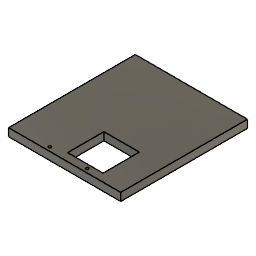
Full (Autodesk Fusion 360 archive; units mm, degrees)
design "rightside"
Autodesk Fusion 360 part; units mm, degrees
sketch "Skizze1" plane through (0, 0, 0) normal (0, 0, 1) x (1, 0, 0)
  line L0 (0, 0) -> (127, 0)
  line L1 (127, 0) -> (127, 143.5)
  line L2 (127, 143.5) -> (0, 143.5)
  line L3 (0, 143.5) -> (0, 0)
  line L4 (98, 50) -> (58, 50)
  line L5 (58, 50) -> (58, 9)
  line L6 (58, 9) -> (98, 9)
  line L7 (98, 9) -> (98, 50)
  circle A0 centre (84.6667, 4.5) radius 1.5
  circle A1 centre (42.3337, 4.5) radius 1.5
  dimension "d1" = 127
  dimension "d2" = 143.5
  dimension "d3" = 40
  dimension "d4" = 29
  dimension "d5" = 50
  dimension "d6" = 41
  dimension "d7" = 3
  dimension "d8" = 4.5
  dimension "d9" = 42.3333
  dimension "d10" = 3
  constraint horizontal L0
  constraint vertical L1
  constraint horizontal L2
  constraint vertical L3
  constraint coincident L0.start L3.end
  constraint perpendicular L3 L4
  constraint perpendicular L4 L5
  constraint perpendicular L5 L6
  constraint perpendicular L4 L7
  measures "d1" distance of L0.start L0.end
  measures "d2" distance of L0.start L2.end
  measures "d3" distance of L4.start L4.end
  measures "d4" distance of L1 L4.start
  measures "d5" distance of L0 L4
  measures "d6" distance of L4.end L5.end
  measures "d7" diameter of A0
  measures "d8" distance of L0 A0.centre
  measures "d9" distance of L1 A0.centre
  measures "d10" diameter of A1
extrude "Extrusion1" add sketch "Skizze1" along normal blind 9
equation "d5 = 41 mm + 9 mm"
equation "d8 = ( 9 / 2 ) * 1 mm"
equation "d9 = ( 127 / 3 ) * 1 mm"

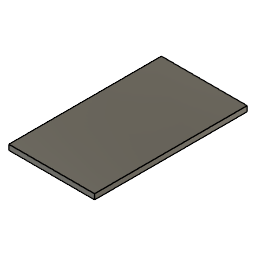
design "Top"
Autodesk Fusion 360 part; units mm, degrees
sketch "Skizze1" plane through (0, 0, 0) normal (0, 0, 1) x (1, 0, 0)
  line L0 (0, 0) -> (145, 0)
  line L1 (145, 0) -> (145, 258)
  line L2 (145, 258) -> (0, 258)
  line L3 (0, 258) -> (0, 0)
  dimension "d1" = 145
  dimension "d2" = 258
  constraint horizontal L0
  constraint vertical L1
  constraint horizontal L2
  constraint vertical L3
  constraint coincident L0.start L3.end
  measures "d1" distance of L0.start L0.end
  measures "d2" distance of L0.start L2.end
extrude "Extrusion2" add sketch "Skizze1" along normal blind 9
equation "d1 = 127 mm + 9 mm + 9 mm"
equation "d2 = 240 mm + 9 mm + 9 mm"

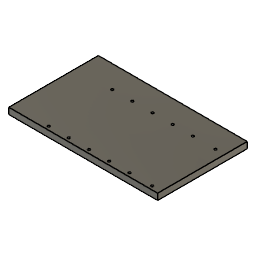
design "screw on plate"
Autodesk Fusion 360 part; units mm, degrees
sketch "Skizze1" plane through (0, 0, 0) normal (0, 0, 1) x (1, 0, 0)
  line L0 (0, 0) -> (-211, 0)
  line L1 (-211, 0) -> (-211, 127)
  line L2 (-211, 127) -> (0, 127)
  line L3 (0, 127) -> (0, 0)
  circle A0 centre (-13, 5) radius 1.625
  circle A1 centre (-13, 95) radius 1.625
  circle A2 centre (-45, 5) radius 1.625
  circle A3 centre (-45, 95) radius 1.625
  circle A4 centre (-73.6, 5) radius 1.625
  circle A5 centre (-73.6, 5) radius 1.625
  circle A6 centre (-102.2, 5) radius 1.625
  circle A7 centre (-130.8, 5) radius 1.625
  circle A8 centre (-159.4, 5) radius 1.625
  circle A9 centre (-73.6, 95) radius 1.625
  circle A10 centre (-102.2, 95) radius 1.625
  circle A11 centre (-159.4, 95) radius 1.625
  circle A12 centre (-130.8, 95) radius 1.625
  dimension "d1" = 211
  dimension "d2" = 127
  dimension "d3" = 3.25
  dimension "d4" = 13
  dimension "d5" = 5
  dimension "d6" = 3.25
  dimension "d7" = 13
  dimension "d8" = 90
  dimension "d9" = 3.25
  dimension "d10" = 32
  dimension "d11" = 3.25
  dimension "d12" = 3.25
  dimension "d13" = 28.6
  dimension "d14" = 3.25
  dimension "d15" = 3.25
  dimension "d16" = 3.25
  dimension "d17" = 3.25
  dimension "d18" = 3.25
  dimension "d19" = 3.25
  dimension "d20" = 3.25
  dimension "d21" = 3.25
  constraint horizontal L0
  constraint vertical L1
  constraint horizontal L2
  constraint vertical L3
  constraint coincident L0.start L3.end
  measures "d1" distance of L0.start L0.end
  measures "d2" distance of L0.start L2.end
  measures "d3" diameter of A0
  measures "d4" distance of L3 A0.centre
  measures "d5" distance of L0 A0.centre
  measures "d6" diameter of A1
  measures "d7" distance of L3 A1.centre
  measures "d8" distance of A0.centre A1.centre
  measures "d9" diameter of A2
  measures "d10" distance of A0.centre A2.centre
  measures "d11" diameter of A3
  measures "d12" diameter of A4
  measures "d13" distance of A2.centre A4.centre
  measures "d14" diameter of A5
  measures "d15" diameter of A6
  measures "d16" diameter of A7
  measures "d17" diameter of A8
  measures "d18" diameter of A9
  measures "d19" diameter of A10
  measures "d20" diameter of A12
  measures "d21" diameter of A11
extrude "Extrusion1" add sketch "Skizze1" along normal blind 9

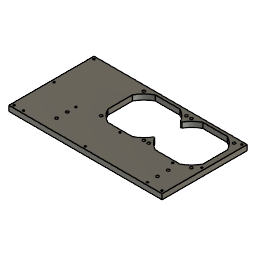
design "back"
Autodesk Fusion 360 part; units mm, degrees
sketch "Skizze1" plane through (0, 0, 0) normal (0, 0, 1) x (1, 0, 0)
  line L0 (258, 143.5) -> (0, 143.5)
  circle A0 centre (229, 39.5) radius 2.25
  circle A1 centre (229, 21.5) radius 2.25
  circle A2 centre (59, 54) radius 1.5
  circle A3 centre (4.5, 4.5) radius 1.5
  circle A4 centre (222, 54) radius 1.5
  circle A5 centre (4.5, 139) radius 1.5
  circle A6 centre (253.5, 4.5) radius 1.5
  circle A7 centre (253.5, 139) radius 1.5
  circle A8 centre (124.5, 4.5) radius 1.5
  circle A9 centre (253.5, 71.75) radius 1.5
  line L1 (0, 143.5) -> (0, 0)
  circle A10 centre (59, 39.5) radius 2.25
  circle A11 centre (20, 4.5) radius 1.5
  circle A12 centre (229, 4.5) radius 1.5
  circle A13 centre (59, 21.5) radius 2.25
  circle A14 centre (4.5, 71.75) radius 1.5
  line L2 (0, 143.5) -> (0, 0) construction
  line L3 (9, 143.5) -> (0, 143.5) construction
  circle A15 centre (133, 54) radius 1.5
  line L4 (0, 0) -> (258, 0)
  line L5 (0, 0) -> (9, 0) construction
  line L6 (258, 0) -> (258, 143.5)
  circle A16 centre (173.1, 134.4) radius 2.25
  arc A17 (210.3507, 143.5) -> (207.6493, 143.5) centre (209, 98.5) ccw construction
  arc A18 (249, 119.1597) -> (229.6597, 138.5) centre (209, 98.5) ccw
  arc A19 (188.3403, 138.5) -> (170.2508, 121.4199) centre (209, 98.5) ccw
  arc A20 (170.2508, 75.5801) -> (188.3403, 58.5) centre (209, 98.5) ccw
  arc A21 (229.6597, 58.5) -> (249, 77.8403) centre (209, 98.5) ccw
  circle A22 centre (244.9, 134.4) radius 2.25
  circle A23 centre (173.1, 62.6) radius 2.25
  circle A24 centre (244.9, 62.6) radius 2.25
  line L7 (188.3403, 138.5) -> (229.6597, 138.5)
  line L8 (249, 119.1597) -> (249, 77.8403)
  line L9 (188.3403, 58.5) -> (229.6597, 58.5)
  arc A25 (149.6597, 58.5) -> (167.7492, 75.5801) centre (129, 98.5) ccw
  arc A26 (167.7492, 121.4199) -> (149.6597, 138.5) centre (129, 98.5) ccw
  line L10 (108.3403, 138.5) -> (149.6597, 138.5)
  arc A27 (108.3403, 138.5) -> (89, 119.1597) centre (129, 98.5) ccw
  line L11 (89, 119.1597) -> (89, 77.8403)
  arc A28 (89, 77.8403) -> (108.3403, 58.5) centre (129, 98.5) ccw
  line L12 (108.3403, 58.5) -> (149.6597, 58.5)
  circle A29 centre (93.1, 134.4) radius 2.25
  circle A30 centre (93.1, 62.6) radius 2.25
  circle A31 centre (164.9, 62.6) radius 2.25
  circle A32 centre (164.9, 134.4) radius 2.25
  arc A33 (167.7492, 121.4199) -> (170.2508, 121.4199) centre (169, 122.1597) ccw
  arc A34 (170.2508, 75.5801) -> (167.7492, 75.5801) centre (169, 74.8403) ccw
  point P0 (253.5, 71.75)
  point P1 (253.5, 139)
  point P2 (253.5, 4.5)
  point P3 (253.5, 4.5)
  point P4 (253.5, 139)
  point P5 (253.5, 71.75)
  dimension "d1" = 143.5
  dimension "d2" = 258
  dimension "d6" = 18
  dimension "d7" = 4.5
  dimension "d8" = 4.5
  dimension "d9" = 4.5
  dimension "d10" = 4.5
  dimension "d11" = 3
  dimension "d12" = 3
  dimension "d13" = 3
  dimension "d14" = 3
  dimension "d15" = 3
  dimension "d22" = 20
  dimension "d24" = 209
  dimension "d26" = 104.5
  dimension "d27" = 3
  dimension "d28" = 3
  dimension "d29" = 3
  dimension "d30" = 67.25
  dimension "d31" = 9
  dimension "d32" = 67.25
  dimension "d33" = 67.25
  dimension "d34" = 3
  dimension "d35" = 3
  dimension "d36" = 3
  dimension "d37" = 67.25
  dimension "d45" = 2.25
  dimension "d47" = 4.5
  dimension "d48" = 4.5
  dimension "d49" = 4.5
  dimension "d50" = 2.25
  dimension "d51" = 4.5
  dimension "d52" = 4.5
  dimension "d53" = 4.5
  constraint horizontal L4
  constraint vertical L6
  constraint horizontal L0
  constraint vertical L1
  constraint coincident L1.end L2.end
  constraint horizontal L5
  constraint horizontal L3
  constraint vertical L2
  constraint coincident L0 A17.end
  constraint coincident L0 A17.start
  constraint concentric A17 A19
  constraint concentric A18 A19
  constraint concentric A19 A20
  constraint concentric A20 A21
  constraint concentric A26 A27
  constraint concentric A27 A28
  constraint concentric A25 A28
  constraint vertical L11
  constraint perpendicular L10 L11
  constraint tangent A19 A33
  measures "d1" distance of L0.end L1.end
  measures "d2" distance of L4.end L1.end
  measures "d6" distance of A13.centre A10.centre
  measures "d7" diameter of A10
  measures "d8" diameter of A13
  measures "d9" diameter of A0
  measures "d10" diameter of A1
  measures "d11" diameter of A15
  measures "d12" diameter of A2
  measures "d13" diameter of A4
  measures "d14" diameter of A11
  measures "d15" diameter of A8
  measures "d22" distance of A11.centre L1
  measures "d24" distance of A12.centre A11.centre
  measures "d26" distance of A8.centre A11.centre
  measures "d27" diameter of A6
  measures "d28" diameter of A7
  measures "d29" diameter of A9
  measures "d30" distance of P5 P1
  measures "d31" distance of L1.end L5.end
  measures "d32" distance of P4 P5
  measures "d33" distance of P5 P4
  measures "d34" diameter of A3
  measures "d35" diameter of A5
  measures "d36" diameter of A14
  measures "d37" distance of A5.centre A14.centre
  measures "d45" radius of A16
  measures "d47" diameter of A22
  measures "d48" diameter of A23
  measures "d49" diameter of A24
  measures "d50" radius of A29
  measures "d51" diameter of A32
  measures "d52" diameter of A30
  measures "d53" diameter of A31
extrude "Extrusion1" add sketch "Skizze1" along normal blind 9

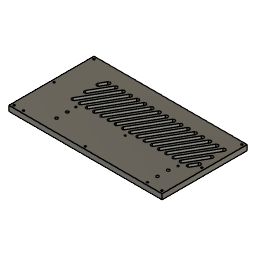
design "front"
Autodesk Fusion 360 part; units mm, degrees
sketch "Skizze1" plane through (0, 0, 0) normal (0, 0, 1) x (1, 0, 0)
  circle A0 centre (229, 39.5) radius 2.25
  circle A1 centre (253.5, 4.5) radius 1.5
  arc A2 (248.408, 114.5) -> (243.2118, 117.5) centre (245.8099, 116) ccw
  line L0 (61.1718, 117.5) -> (42.9969, 86.0202)
  line L1 (121.8518, 117.5) -> (91.5409, 65)
  arc A3 (236.272, 114.5) -> (231.0758, 117.5) centre (233.6739, 116) ccw
  line L2 (243.2118, 117.5) -> (212.9009, 65)
  line L3 (0, 0) -> (258, 0)
  line L4 (218.9398, 117.5) -> (188.6289, 65)
  line L5 (187.728, 114.5) -> (157.4171, 62)
  line L6 (212, 114.5) -> (181.6891, 62)
  line L7 (194.6678, 117.5) -> (164.3569, 65)
  circle A4 centre (231, 54) radius 1.5
  circle A5 centre (229, 21.5) radius 2.25
  arc A6 (212, 114.5) -> (206.8038, 117.5) centre (209.4019, 116) ccw
  line L8 (231.0758, 117.5) -> (200.7649, 65)
  line L9 (206.8038, 117.5) -> (176.4929, 65)
  arc A7 (199.864, 114.5) -> (194.6678, 117.5) centre (197.2659, 116) ccw
  line L10 (258, 0) -> (258, 143.5)
  line L11 (85.4438, 117.5) -> (55.1329, 65)
  arc A8 (187.728, 114.5) -> (182.5318, 117.5) centre (185.1299, 116) ccw
  line L12 (199.864, 114.5) -> (169.5531, 62)
  line L13 (73.3078, 117.5) -> (42.9969, 65)
  circle A9 centre (229, 4.5) radius 1.5
  line L14 (0, 143.5) -> (0, 0)
  line L15 (248.408, 114.5) -> (218.0971, 62)
  line L16 (242.3701, 62) -> (248.5981, 72.7872)
  line L17 (109.7158, 117.5) -> (79.4049, 65)
  circle A10 centre (253.5, 139) radius 1.5
  arc A11 (224.136, 114.5) -> (218.9398, 117.5) centre (221.5379, 116) ccw
  arc A12 (102.776, 114.5) -> (97.5798, 117.5) centre (100.1779, 116) ccw
  arc A13 (248.5981, 93.8074) -> (243.4019, 96.8074) centre (246, 95.3074) ccw
  arc A14 (200.7649, 65) -> (205.9611, 62) centre (203.363, 63.5) ccw
  line L18 (102.776, 114.5) -> (72.4651, 62)
  arc A15 (127.9489, 65) -> (133.1451, 62) centre (130.547, 63.5) ccw
  line L19 (146.1238, 117.5) -> (115.8129, 65)
  arc A16 (164.3569, 65) -> (169.5531, 62) centre (166.955, 63.5) ccw
  line L20 (175.592, 114.5) -> (145.2811, 62)
  line L21 (139.184, 114.5) -> (108.8731, 62)
  arc A17 (127.048, 114.5) -> (121.8518, 117.5) centre (124.4499, 116) ccw
  line L22 (114.912, 114.5) -> (84.6011, 62)
  arc A18 (140.0849, 65) -> (145.2811, 62) centre (142.683, 63.5) ccw
  line L23 (258, 143.5) -> (0, 143.5)
  arc A19 (175.592, 114.5) -> (170.3958, 117.5) centre (172.9939, 116) ccw
  arc A20 (115.8129, 65) -> (121.0091, 62) centre (118.411, 63.5) ccw
  arc A21 (176.4929, 65) -> (181.6891, 62) centre (179.091, 63.5) ccw
  line L24 (182.5318, 117.5) -> (152.2209, 65)
  line L25 (170.3958, 117.5) -> (140.0849, 65)
  arc A22 (103.6769, 65) -> (108.8731, 62) centre (106.275, 63.5) ccw
  arc A23 (152.2209, 65) -> (157.4171, 62) centre (154.819, 63.5) ccw
  line L26 (158.2598, 117.5) -> (127.9489, 65)
  line L27 (133.9878, 117.5) -> (103.6769, 65)
  circle A24 centre (124.5, 4.5) radius 1.5
  arc A25 (114.912, 114.5) -> (109.7158, 117.5) centre (112.3139, 116) ccw
  arc A26 (139.184, 114.5) -> (133.9878, 117.5) centre (136.5859, 116) ccw
  line L28 (163.456, 114.5) -> (133.1451, 62)
  arc A27 (151.32, 114.5) -> (146.1238, 117.5) centre (148.7219, 116) ccw
  line L29 (151.32, 114.5) -> (121.0091, 62)
  arc A28 (163.456, 114.5) -> (158.2598, 117.5) centre (160.8579, 116) ccw
  circle A29 centre (142, 54) radius 1.5
  arc A30 (225.0379, 65) -> (230.2341, 62) centre (227.636, 63.5) ccw
  arc A31 (188.6289, 65) -> (193.8251, 62) centre (191.227, 63.5) ccw
  line L30 (237.1739, 65) -> (243.4019, 75.7872)
  arc A32 (237.1739, 65) -> (242.3701, 62) centre (239.772, 63.5) ccw
  line L31 (230.2341, 62) -> (248.5981, 93.8074)
  line L32 (225.0379, 65) -> (243.4019, 96.8074)
  arc A33 (212.9009, 65) -> (218.0971, 62) centre (215.499, 63.5) ccw
  arc A34 (248.5981, 72.7872) -> (243.4019, 75.7872) centre (246, 74.2872) ccw
  circle A35 centre (253.5, 71.75) radius 1.5
  line L33 (127.048, 114.5) -> (96.7371, 62)
  line L34 (224.136, 114.5) -> (193.8251, 62)
  line L35 (236.272, 114.5) -> (205.9611, 62)
  arc A36 (90.64, 114.5) -> (85.4438, 117.5) centre (88.0419, 116) ccw
  arc A37 (91.5409, 65) -> (96.7371, 62) centre (94.139, 63.5) ccw
  line L36 (66.368, 114.5) -> (48.1931, 83.0202)
  line L37 (78.504, 114.5) -> (48.1931, 62)
  circle A38 centre (4.5, 139) radius 1.5
  circle A39 centre (4.5, 4.5) radius 1.5
  arc A40 (78.504, 114.5) -> (73.3078, 117.5) centre (75.9059, 116) ccw
  arc A41 (66.368, 114.5) -> (61.1718, 117.5) centre (63.7699, 116) ccw
  line L38 (54.232, 114.5) -> (48.1931, 104.0403)
  arc A42 (42.9969, 86.0202) -> (48.1931, 83.0202) centre (45.595, 84.5202) ccw
  line L39 (97.5798, 117.5) -> (67.2689, 65)
  line L40 (90.64, 114.5) -> (60.3291, 62)
  line L41 (49.0358, 117.5) -> (42.9969, 107.0403)
  arc A43 (42.9969, 107.0403) -> (48.1931, 104.0403) centre (45.595, 105.5403) ccw
  arc A44 (54.232, 114.5) -> (49.0358, 117.5) centre (51.6339, 116) ccw
  circle A45 centre (59, 54) radius 1.5
  arc A46 (55.1329, 65) -> (60.3291, 62) centre (57.731, 63.5) ccw
  circle A47 centre (4.5, 71.75) radius 1.5
  arc A48 (79.4049, 65) -> (84.6011, 62) centre (82.003, 63.5) ccw
  circle A49 centre (59, 21.5) radius 2.25
  arc A50 (67.2689, 65) -> (72.4651, 62) centre (69.867, 63.5) ccw
  arc A51 (42.9969, 65) -> (48.1931, 62) centre (45.595, 63.5) ccw
  circle A52 centre (59, 39.5) radius 2.25
  circle A53 centre (20, 4.5) radius 1.5
  point P0 (253.5, 71.75)
  point P1 (253.5, 139)
  point P2 (253.5, 4.5)
  point P3 (253.5, 4.5)
  point P4 (253.5, 139)
  point P5 (253.5, 71.75)
  dimension "d3" = 12.136
  dimension "d4" = 0
  dimension "d7" = 12.136
  dimension "d8" = 0
  dimension "d9" = 143.5
  dimension "d10" = 258
  dimension "d14" = 18
  dimension "d15" = 4.5
  dimension "d16" = 4.5
  dimension "d17" = 4.5
  dimension "d18" = 4.5
  dimension "d19" = 3
  dimension "d20" = 3
  dimension "d21" = 3
  dimension "d22" = 3
  dimension "d23" = 3
  dimension "d30" = 20
  dimension "d32" = 209
  dimension "d34" = 104.5
  dimension "d35" = 3
  dimension "d36" = 3
  dimension "d37" = 3
  dimension "d38" = 67.25
  dimension "d40" = 67.25
  dimension "d41" = 67.25
  dimension "d42" = 3
  dimension "d43" = 3
  dimension "d44" = 3
  dimension "d45" = 67.25
  dimension "d46" = 3
  dimension "d51" = 27
  dimension "d52" = 116
  constraint horizontal L3
  constraint vertical L10
  constraint horizontal L23
  constraint vertical L14
  constraint coincident L3.start L14.end
  constraint tangent A13 L32
  constraint tangent A13 L31
  constraint tangent L30 A34
  constraint tangent L16 A34
  constraint tangent L41 A43
  constraint tangent L38 A43
  constraint parallel L38 L41
  constraint tangent L0 A42
  constraint tangent L36 A42
  constraint tangent L13 A51
  constraint tangent L37 A51
  constraint tangent L13 A40
  constraint tangent L37 A40
  measures "d9" distance of L14.start L3.start
  measures "d10" distance of L3.end L3.start
  measures "d14" distance of A49.centre A52.centre
  measures "d15" diameter of A52
  measures "d16" diameter of A49
  measures "d17" diameter of A0
  measures "d18" diameter of A5
  measures "d19" diameter of A29
  measures "d20" diameter of A45
  measures "d21" diameter of A4
  measures "d22" diameter of A53
  measures "d23" diameter of A24
  measures "d30" distance of A53.centre L14
  measures "d32" distance of A9.centre A53.centre
  measures "d34" distance of A24.centre A53.centre
  measures "d35" diameter of A1
  measures "d36" diameter of A10
  measures "d37" diameter of A35
  measures "d38" distance of P5 P1
  measures "d40" distance of P4 P5
  measures "d41" distance of P5 P4
  measures "d42" diameter of A39
  measures "d43" diameter of A38
  measures "d44" diameter of A47
  measures "d45" distance of A38.centre A47.centre
  measures "d46" radius of A51
  measures "d51" distance of A4.centre L10
  measures "d52" distance of A29.centre L10
extrude "Extrusion1" add sketch "Skizze1" along normal blind 9

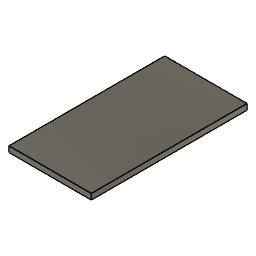
design "Bottom"
Autodesk Fusion 360 part; units mm, degrees
sketch "Skizze1" plane through (0, 0, 0) normal (0, 0, 1) x (1, 0, 0)
  line L0 (0, 0) -> (127, 0)
  line L1 (127, 0) -> (127, 240)
  line L2 (127, 240) -> (0, 240)
  line L3 (0, 240) -> (0, 0)
  dimension "d1" = 127
  dimension "d2" = 240
  constraint horizontal L0
  constraint vertical L1
  constraint horizontal L2
  constraint vertical L3
  constraint coincident L0.start L3.end
  measures "d1" distance of L0.start L0.end
  measures "d2" distance of L0.start L2.end
extrude "Extrusion1" add sketch "Skizze1" along normal blind 9

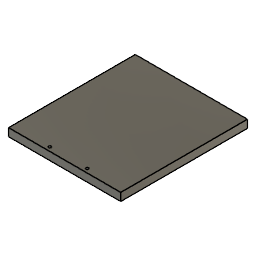
design "leftside"
Autodesk Fusion 360 part; units mm, degrees
sketch "Skizze1" plane through (0, 0, 0) normal (0, 0, 1) x (1, 0, 0)
  line L0 (127, 0) -> (127, 143.5)
  line L1 (0, 143.5) -> (0, 0)
  line L2 (0, 0) -> (127, 0)
  circle A0 centre (84.6667, 4.5) radius 1.5
  circle A1 centre (42.3337, 4.5) radius 1.5
  line L3 (127, 143.5) -> (0, 143.5)
  dimension "d1" = 127
  dimension "d2" = 143.5
  dimension "d7" = 3
  dimension "d8" = 4.5
  dimension "d9" = 42.3333
  dimension "d10" = 3
  constraint horizontal L2
  constraint vertical L0
  constraint horizontal L3
  constraint vertical L1
  constraint coincident L1.end L2.start
  measures "d1" distance of L0.start L1.end
  measures "d2" distance of L1.end L1.start
  measures "d7" diameter of A0
  measures "d8" distance of A0.centre L2
  measures "d9" distance of A0.centre L0
  measures "d10" diameter of A1
extrude "Extrusion1" add sketch "Skizze1" along normal blind 9
